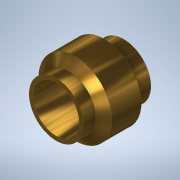
# Autodesk Inventor part: MINI-olive
Saved by Autodesk Inventor 2021 (Build 250183000, 183)
## iProperties
Created: 2019-10-03
Material: Všeobecné
Document SubType Name: Modeling
Density: 1 g/cm^3
Appearance: Mosaz – leštěná
Project: ORIGINAL PRUSA MINI
Authority: Ing. Robert Turinský
Company: Prusa Development a.s.
Author: Ing. Robert Turinský
Revision Number: R4
Autodesk Inventor part; units mm, degrees
ref_plane "YZ Plane" through (0, 0, 0) normal (1, 0, 0) x (0, 1, 0)
ref_plane "XZ Plane" through (0, 0, 0) normal (0, 1, 0) x (-1, 0, 0)
ref_plane "XY Plane" through (0, 0, 0) normal (0, 0, 1) x (1, 0, 0)
sketch "Náčrt1" plane through (0, 0, 0) normal (0, 1, 0) x (-1, 0, 0)
  line L0 (3.9, 0) -> (-0.65, 0) projected
  line L1 (0, -1.2) -> (0, 7.2) projected
  line L2 (2.05, 0) -> (2.05, 6)
  line L3 (2.05, 6) -> (2.4, 6)
  line L4 (2.4, 6) -> (2.4, 4.9)
  line L5 (2.4, 4.9) -> (3.25, 4.3048)
  line L6 (3.25, 4.3048) -> (3.25, 1.6952)
  line L7 (3.25, 1.6952) -> (2.4, 1.1)
  line L8 (2.4, 1.1) -> (2.4, 0)
  line L9 (2.4, 0) -> (2.05, 0)
  point P0 (0, 0)
  dimension "d0" = 4.1
  dimension "d1" = 4.8
  dimension "d2" = 6
  dimension "d3" = 6.5
  dimension "d4" = 1.1
  dimension "d6" = 125
  constraints: 16 end point, 4 point on line, 2 equal length, 2 perpendicular, 1 collinear, 1 parallel, 1 vertical
  measures "d0" diameter of L2 L1
  measures "d1" diameter of L4 L1
  measures "d2" distance of L2.start L2.end
  measures "d3" diameter of L6 L1
  measures "d4" distance of L3.end L4.end
  measures "d6" angle of L6 L7
revolve "Rotace1" add sketch "Náčrt1" angle 360 about axis through (0, 0, -10) along (0, 0, 1)
